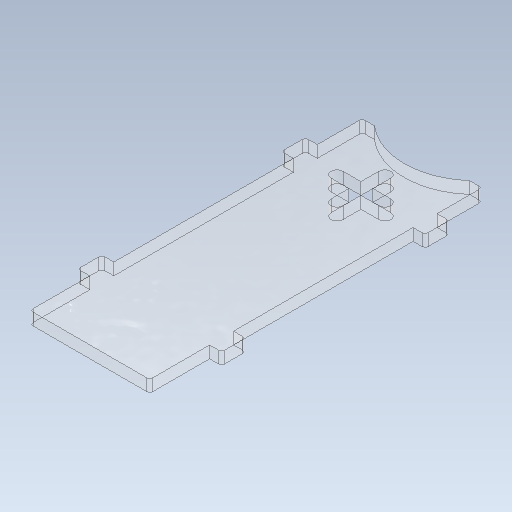
# Autodesk Inventor part: Laser-Slot-Top
Saved by Autodesk Inventor 2021 (Build 250183000, 183)
## iProperties
Created: 2020-07-21
Part Number: Laser-Slot-Top
Material: Acrylic, Clear
Document SubType Name: Modeling
Designer: lucas
Density: 1.19 g/cm^3
Appearance: Transparent - Clear
Project: 4Wire-Laser
Author: lucas
Revision Number: RLS_001
Autodesk Inventor part; units mm, degrees
ref_plane "YZ Plane" through (0, 0, 0) normal (1, 0, 0) x (0, 1, 0)
ref_plane "XZ Plane" through (0, 0, 0) normal (0, 1, 0) x (-1, 0, 0)
ref_plane "XY Plane" through (0, 0, 0) normal (0, 0, 1) x (1, 0, 0)
sketch "Sketch1" plane through (0, 0, 0) normal (0, 1, 0) x (-1, 0, 0)
  line L0 (9.5, 29) -> (-9.5, 29)
  line L1 (-9.5, -26.5) -> (-7.9373, -26.5)
  line L2 (10, 0) -> (10, 15)
  line L3 (10, 15) -> (11.5, 15)
  line L4 (12, 15.5) -> (12, 18.5)
  line L5 (11.5, 19) -> (10, 19)
  line L6 (10, 0) -> (10, -15)
  line L7 (10, -15) -> (11.5, -15)
  line L8 (12, -15.5) -> (12, -18.5)
  line L9 (11.5, -19) -> (10, -19)
  line L10 (-10, 0) -> (-10, 15)
  line L11 (-10, 15) -> (-11.5, 15)
  line L12 (-12, 15.5) -> (-12, 18.5)
  line L13 (-11.5, 19) -> (-10, 19)
  line L14 (-10, 0) -> (-10, -15)
  line L15 (-10, -15) -> (-11.5, -15)
  line L16 (-12, -15.5) -> (-12, -18.5)
  line L17 (-11.5, -19) -> (-10, -19)
  line L18 (10, 19) -> (10, 28.5)
  line L19 (10, -19.5) -> (10, -19)
  line L20 (10, -15) -> (10, 15)
  line L21 (-10, -19) -> (-10, -19.5)
  line L22 (-10, 28.5) -> (-10, 19)
  line L23 (-10, 15) -> (-10, -15)
  arc A0 (11.5, 15) -> (12, 15.5) centre (11.5, 15.5) ccw
  arc A1 (12, 18.5) -> (11.5, 19) centre (11.5, 18.5) ccw
  arc A2 (-11.5, 19) -> (-12, 18.5) centre (-11.5, 18.5) ccw
  arc A3 (-12, 15.5) -> (-11.5, 15) centre (-11.5, 15.5) ccw
  arc A4 (12, -15.5) -> (11.5, -15) centre (11.5, -15.5) ccw
  arc A5 (11.5, -19) -> (12, -18.5) centre (11.5, -18.5) ccw
  arc A6 (-11.5, -15) -> (-12, -15.5) centre (-11.5, -15.5) ccw
  arc A7 (-12, -18.5) -> (-11.5, -19) centre (-11.5, -18.5) ccw
  line L24 (0, -26.5) -> (0, -35.5) construction
  arc A8 (7.9373, -26.5) -> (-7.9373, -26.5) centre (0, -35.5) ccw
  arc A9 (10, 28.5) -> (9.5, 29) centre (9.5, 28.5) ccw
  arc A10 (-9.5, 29) -> (-10, 28.5) centre (-9.5, 28.5) ccw
  line L25 (7.9373, -26.5) -> (9.5, -26.5)
  line L26 (-7.9373, -26.5) -> (7.9373, -26.5) construction
  line L27 (0, -26.5) -> (0, -26.5) construction
  line L28 (10, -19.5) -> (10, -26)
  line L29 (9.5, -26.5) -> (9.5, -26.5)
  line L30 (-10, -19.5) -> (-10, -26)
  line L31 (-9.5, -26.5) -> (-9.5, -26.5)
  arc A11 (9.5, -26.5) -> (10, -26) centre (9.5, -26) ccw
  arc A12 (-10, -26) -> (-9.5, -26.5) centre (-9.5, -26) ccw
  line L32 (0, 29) -> (0, 29) construction
  point P0 (0, 0)
  point P1 (12, 15)
  point P2 (12, 19)
  point P3 (12, -15)
  point P4 (12, -19)
  point P5 (-12, 15)
  point P6 (-12, 19)
  point P7 (-12, -15)
  point P8 (-12, -19)
  point P9 (-10, -26.5)
  dimension "d2" = 15
  dimension "d3" = 2
  dimension "d4" = 4
  dimension "d5" = 15
  dimension "d6" = 4
  dimension "d7" = 15
  dimension "d8" = 2
  dimension "d9" = 4
  dimension "d10" = 15
  dimension "d11" = 4
  dimension "d12" = 0.5
  dimension "d13" = 9
  dimension "d14" = 12
  dimension "d15" = 0.5
  dimension "d26" = 0
  dimension "d27" = 0.5
  dimension "d28" = 0
  constraints: 66 end point, 26 perpendicular, 26 point on circle, 24 tangent, 22 point on line, 13 centre point, 12 parallel, 9 equal radius, 5 coincident, 3 midpoint, 3 vertical, 1 collinear, 1 horizontal
  measures "d2" distance of L2.start L2.end
  measures "d3" distance of L2.end point (12, 15)
  measures "d4" distance of point (12, 15) point (12, 19)
  measures "d5" distance of L2.start L6.end
  measures "d6" distance of point (12, -15) point (12, -19)
  measures "d7" distance of L10.start L10.end
  measures "d8" distance of L10.end point (-12, 15)
  measures "d9" distance of point (-12, 15) point (-12, 19)
  measures "d10" distance of L10.start L14.end
  measures "d11" distance of point (-12, -15) point (-12, -19)
  measures "d12" radius of A0
  measures "d13" distance of L24.start L24.end
  measures "d14" radius of A8
  measures "d15" radius of A9
  measures "d26" distance of L24.start L27.end
  measures "d27" radius of A11
  measures "d28" distance of L32.start L32.end
extrude "Extrusion1" add sketch "Sketch1" along normal blind 2
sketch "Sketch2" plane through (0, 2, 0) normal (0, 1, 0) x (1, 0, 0)
  line L0 (-4, 16.2872) -> (4, 16.2872) construction
  line L1 (-4, 15.2872) -> (4, 15.2872)
  line L2 (4, 17.2872) -> (-4, 17.2872)
  arc A0 (-4, 17.2872) -> (-4, 15.2872) centre (-4, 16.2872) ccw
  arc A1 (4, 15.2872) -> (4, 17.2872) centre (4, 16.2872) ccw
  line L3 (0, 20.2872) -> (0, 12.2872) construction
  line L4 (-1, 20.2872) -> (-1, 12.2872)
  line L5 (1, 12.2872) -> (1, 20.2872)
  arc A2 (1, 20.2872) -> (-1, 20.2872) centre (0, 20.2872) ccw
  arc A3 (-1, 12.2872) -> (1, 12.2872) centre (0, 12.2872) ccw
  line L6 (0, 16.2872) -> (0, 21.2872) construction
  point P0 (0, 0)
  point P1 (-1, 15.2872)
  point P2 (1, 15.2872)
  point P3 (1, 17.2872)
  point P4 (-1, 17.2872)
  point P5 (0, 21.2872)
  dimension "d18" = 4
  dimension "d19" = 2
  dimension "d20" = 4
  dimension "d21" = 2
  dimension "d29" = 5
  constraints: 18 end point, 10 point on circle, 8 tangent, 4 centre point, 2 midpoint, 2 parallel, 1 coincident, 1 horizontal, 1 perpendicular
  measures "d18" distance of L6.start L0.end
  measures "d19" diameter of A1
  measures "d20" distance of L6.start L3.end
  measures "d21" diameter of A3
  measures "d29" distance of L6.start L6.end
extrude "Extrusion2" cut sketch "Sketch2" against normal blind 2
body "Solid1"
